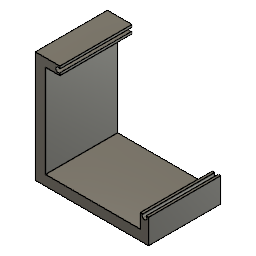
Brace v3 (Autodesk Fusion 360 design; units mm, degrees)
Autodesk Fusion 360 part; units mm, degrees
sketch "Sketch1" plane through (0, 0, 0) normal (0, 1, 0) x (1, 0, 0)
  line L0 (0, 0) -> (44, 0)
  line L1 (44, 0) -> (44, -35)
  line L2 (44, -35) -> (0, -35)
  line L3 (0, -35) -> (0, 0)
  line L4 (0, 0) -> (-5, 0)
  line L5 (0, -35) -> (-5, -35)
  line L6 (-5, -35) -> (-5, 0)
  dimension "d1" = 44
  dimension "d2" = 35
  dimension "d3" = 5
  dimension "d4" = 5
  constraint coincident L0.start L3.end
  constraint perpendicular L1 L2
  constraint perpendicular L0 L3
  constraint perpendicular L4 L6
  measures "d1" distance of L0.start L0.end
  measures "d2" distance of L0.end L1.end
  measures "d3" distance of L0.start L4.end
  measures "d4" distance of L2.end L5.end
extrude "Extrude1" add sketch "Sketch1" along normal blind 49 contours L3 L4 L5 L6 makes body 1
sketch "Sketch2" plane through (0, 0, 0) normal (0, 1, 0) x (1, 0, 0)
  line L0 (0, 0) -> (44, 0)
  line L1 (44, 0) -> (44, -35)
  line L2 (44, -35) -> (0, -35)
  line L3 (0, -35) -> (0, 0)
  dimension "d7" = 44
  constraint horizontal L0
  constraint vertical L1
  constraint horizontal L2
  constraint vertical L3
  constraint coincident L0.start L3.end
  measures "d7" distance of L0.start L0.end
extrude "Extrude2" add sketch "Sketch2" against normal blind 2 separate body makes body 2
extrude "Extrude3" add 1 faces at (-3.3333, 0, 11.6667) along direction (0, -1, 0) blind 2 on bodies 1 bodies 1 2
extrude "Extrude4" cut 1 faces at (-5, 15, 23.3333) along direction (1, 0, 0) blind 3 on bodies 1 bodies 1
extrude "Extrude5" add 1 faces at (14, -2, 11.6667) along direction (0, -1, 0) blind 3 on bodies 1 bodies 1
extrude "Extrude6" add 1 faces at (-2, 13, 11.6667) along direction (-1, 0, 0) blind 3 on bodies 1 bodies 1
sketch "Sketch3" plane through (0, 0, 0) normal (0, 0, 1) x (1, 0, 0)
  line L0 (40, 0) -> (44, 0)
  line L1 (0, 49) -> (7, 49)
  line L2 (7.3361, 44.9497, 0.0019) -> (7.3361, 48.9497, 0.0019)
  line L3 (9.3361, 48.9497, 0.0019) -> (7.3361, 48.9497, 0.0019)
  line L4 (0.0061, 48.9497, 0.0019) -> (0.0061, 44.9497, 0.0019)
  line L5 (0.0061, 44.9497, 0.0019) -> (7.3361, 44.9497, 0.0019)
  line L6 (7.3361, 44.9497, 0.0019) -> (7.3361, 48.9497, 0.0019)
  line L7 (9.3361, 44.9497, 0.0019) -> (9.3361, 48.9497, 0.0019)
  line L8 (0.0061, 44.9497, 0.0019) -> (7.3361, 44.9497, 0.0019)
  line L9 (7.3361, 48.9497, 0.0019) -> (0.0061, 48.9497, 0.0019)
  line L10 (7.3361, 48.9497, 0.0019) -> (7.3361, 44.9497, 0.0019)
  circle A0 through (9.6661, 46.9497, 0.0019) (7.9186, 47.9586, 0.0019) (7.9186, 45.9408, 0.0019)
  circle A1 through (9.6661, 46.9497, 0.0019) (7.9186, 47.9586, 0.0019) (7.9186, 45.9408, 0.0019)
  line L11 (9.3361, 44.9497, 0.0019) -> (9.3361, 48.9497, 0.0019)
  line L12 (7.3361, 48.9497, 0.0019) -> (0.0061, 48.9497, 0.0019)
  line L13 (7.3361, 48.9497, 0.0019) -> (7.3361, 44.9497, 0.0019)
  line L14 (7.3361, 44.9497, 0.0019) -> (9.3361, 44.9497, 0.0019)
  line L15 (7.3361, 44.9497, 0.0019) -> (7.3361, 48.9497, 0.0019)
  line L16 (9.3361, 48.9497, 0.0019) -> (7.3361, 48.9497, 0.0019)
  line L17 (7.3361, 44.9497, 0.0019) -> (9.3361, 44.9497, 0.0019)
  line L18 (7.3361, 44.9497, 0.0019) -> (9.3361, 44.9497, 0.0019)
  line L19 (7.3361, 48.9497, 0.0019) -> (0.0061, 48.9497, 0.0019)
  line L20 (0.0061, 44.9497, 0.0019) -> (7.3361, 44.9497, 0.0019)
  line L21 (7.3361, 48.9497, 0.0019) -> (7.3361, 44.9497, 0.0019)
  line L22 (9.3361, 44.9497, 0.0019) -> (9.3361, 48.9497, 0.0019)
  circle A2 through (9.6661, 46.9497, 0.0019) (7.9186, 47.9586, 0.0019) (7.9186, 45.9408, 0.0019)
  line L23 (9.3361, 48.9497, 0.0019) -> (7.3361, 48.9497, 0.0019)
  line L24 (40, 0) -> (0, 0)
  line L25 (0, 0) -> (0, 45)
  line L26 (40, 0) -> (0, 0)
  line L27 (0, 0) -> (0, 45)
  line L28 (44, 0) -> (40, 0)
  line L29 (40, 0) -> (40, 5)
  line L30 (40, 5) -> (44, 5)
  line L31 (44, 5) -> (44, 0)
  line L32 (40, 5) -> (44, 5)
  line L33 (44, 5) -> (44, 7)
  line L34 (44, 7) -> (40, 7)
  line L35 (40, 7) -> (40, 5)
  circle A3 centre (42, 6.165) radius 1.165
  point P0 (44, 0)
  point P1 (44, 0)
  point P2 (0.0061, 44.9497)
  dimension "d77" = 5
  dimension "d78" = 4
  dimension "d79" = 2
  dimension "d80" = 2.33
  constraint coincident P0 L0.end
  constraint coincident L24.end L25.start
  constraint perpendicular L24 L25
  constraint horizontal L26
  constraint vertical L27
  constraint horizontal L28
  constraint vertical L29
  constraint horizontal L30
  constraint vertical L31
  constraint coincident P1 P0
  constraint horizontal L32
  constraint vertical L33
  constraint horizontal L34
  constraint vertical L35
  measures "d77" distance of P1 L30.end
  measures "d78" distance of L29.end L30.end
  measures "d79" distance of L29.end L34.end
  measures "d80" diameter of A3
extrude "Extrude9" add sketch "Sketch3" along normal blind 35 contours L0 L28 L29 L30 L31 L32 | L30 L32 L34 L35 A3 | L30 L32 L33 L34 A3 bodies 1
extrude "Extrude10" cut 1 faces at (0, 16.3333, 23.3333) along direction (-1, 0, 0) blind 1 on bodies 1 bodies 1
extrude "Extrude11" add 1 faces at (-5, 13, 11.6667) along direction (-1, 0, 0) blind 1 on bodies 1 bodies 1
extrude "Extrude13" add 1 faces at (-6, 13, 11.6667) along direction (-1, 0, 0) blind 5 on bodies 1 bodies 1
extrude "Extrude14" cut 1 faces at (-1, 16.3333, 23.3333) along direction (-1, 0, 0) blind 5 on bodies 1 bodies 1
sketch "Sketch5" plane through (0, 0, 0) normal (0, 0, 1) x (1, 0, 0)
  line L0 (1, 49) -> (-1, 49)
  line L1 (1, 45) -> (1, 49)
  line L2 (-1, 45) -> (1, 45)
  circle A0 centre (0.165, 47) radius 1.165
  line L3 (-1, 49) -> (-1, 45)
  line L4 (-6, 49) -> (-1, 49)
  line L5 (-6, 45) -> (-6, 49)
  line L6 (-6, 49) -> (-6, 45)
  line L7 (-1, 45) -> (-6, 45)
  line L8 (-1, 49) -> (-1, 45)
  point P0 (-6, 49)
  point P1 (-6, 45)
  point P2 (-6, 45)
  dimension "d87" = 5
  dimension "d88" = 4
  dimension "d89" = 2
  dimension "d90" = 2.33
  constraint coincident P2 P1
  measures "d87" distance of L2.start P2
  measures "d88" distance of L2.start L0.end
  measures "d89" distance of L0.start L0.end
  measures "d90" diameter of A0
extrude "Extrude15" add sketch "Sketch5" along normal blind 35 contours L0 L1 A0 L3 L8 | L3 L4 L5 L6 L7 L8 | L1 L2 A0 L3 L8 bodies 1
extrude "Extrude12" [suppressed]
extrude "Extrude7" [suppressed]
sketch "Sketch4" plane through (0, 0, 0) normal (0, 0, 1) x (1, 0, 0)
  line L0 (7.33, 45) -> (7.33, 49)
  line L1 (9.33, 49) -> (7.33, 49)
  line L2 (0, 49) -> (0, 45)
  line L3 (0, 45) -> (7.33, 45)
  line L4 (7.33, 45) -> (7.33, 49)
  line L5 (9.33, 45) -> (9.33, 49)
  line L6 (0, 45) -> (7.33, 45)
  line L7 (7.33, 49) -> (0, 49)
  line L8 (7.33, 49) -> (7.33, 45)
  circle A0 centre (8.495, 47) radius 1.165
  circle A1 centre (8.495, 47) radius 1.165
  line L9 (9.33, 45) -> (9.33, 49)
  line L10 (7.33, 49) -> (0, 49)
  line L11 (7.33, 49) -> (7.33, 45)
  line L12 (7.33, 45) -> (9.33, 45)
  line L13 (7.33, 45) -> (7.33, 49)
  line L14 (9.33, 49) -> (7.33, 49)
  line L15 (7.33, 45) -> (9.33, 45)
  line L16 (7.33, 45) -> (9.33, 45)
  line L17 (7.33, 49) -> (0, 49)
  line L18 (0, 45) -> (7.33, 45)
  line L19 (7.33, 49) -> (7.33, 45)
  line L20 (9.33, 45) -> (9.33, 49)
  circle A2 centre (8.495, 47) radius 1.165
  line L21 (9.33, 49) -> (7.33, 49)
  point P0 (0, 45)
  dimension "d66" = 7.33
  dimension "d67" = 4
  dimension "d68" = 2
  dimension "d69" = 7.33
  dimension "d70" = 4
  dimension "d71" = 2
  dimension "d72" = 7.33
  dimension "d73" = 4
  dimension "d74" = 2
  constraint coincident P0 L2.end
  constraint perpendicular L13 L17
  constraint perpendicular L2 L6
  constraint tangent A1 L13
  constraint perpendicular L0 L7
  constraint tangent L0 A0
  constraint perpendicular L4 L10
  constraint tangent L4 A2
  measures "d66" distance of L0.start P0
  measures "d67" distance of L0.start L0.end
  measures "d68" distance of L0.end L1.start
  measures "d69" distance of L0.start P0
  measures "d70" distance of L0.start L0.end
  measures "d71" distance of L0.end L1.start
  measures "d72" distance of L0.start P0
  measures "d73" distance of L0.start L0.end
  measures "d74" distance of L0.end L1.start
extrude "Extrude8" [suppressed]
